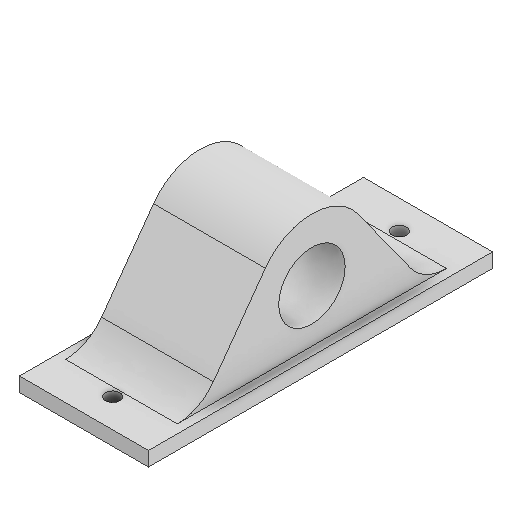
# Autodesk Inventor part: 8P - MainWing Joint
Saved by Autodesk Inventor 2025.1 (Build 291241000, 241)
## iProperties
Category: <PART CATAGORY>
Created: 2024-11-07
Part Number: 8P - MainWing Joint
Material: Generic
Document SubType Name: Modeling
Designer: alptl
Density: 1 g/cm^3
Appearance: Default
Title: <TITLE>
Author: alptl
Revision Number: 1
Autodesk Inventor part; units mm, degrees
ref_plane "YZ Plane" through (0, 0, 0) normal (1, 0, 0) x (0, 1, 0)
ref_plane "XZ Plane" through (0, 0, 0) normal (0, 1, 0) x (-1, 0, 0)
ref_plane "XY Plane" through (0, 0, 0) normal (0, 0, 1) x (1, 0, 0)
sketch "Sketch6" plane through (0, 0, 0) normal (0, 1, 0) x (-1, 0, 0)
  line L0 (22.5, 0) -> (22.5, -60)
  line L1 (22.5, -60) -> (-22.5, -60)
  line L2 (-22.5, -60) -> (-22.5, 0)
  circle A0 centre (0, -50) radius 2.5
  line L3 (-22.5, 0) -> (22.5, 0)
  point P0 (0, 0)
  dimension "d85" = 22.5
  dimension "d86" = 60
  dimension "d87" = 45
  dimension "d89" = 5
  constraints: 8 end point, 3 perpendicular, 1 centre point, 1 coincident
  measures "d85" distance of point (0, 0) L0.start
  measures "d86" distance of L0.start L0.end
  measures "d87" distance of L0.end L1.end
  measures "d89" diameter of A0
extrude "Extrusion3" add sketch "Sketch6" along normal blind 5
mirror "Mirror3" about plane through (-22.5, 0, 0) normal (0, 0, 1) of "Extrusion3"
sketch "Sketch7" plane through (0, 0, -60) normal (1, 0, 0) x (0, 0, -1)
  arc A0 (-43.7585, 36.671) -> (-76.2415, 36.671) centre (-60, 25) ccw
  circle A1 centre (-60, 23.3) radius 11.6
  line L0 (0, 5) -> (-120, 5) projected
  line L1 (-60, 5) -> (-99, 5)
  line L2 (-99, 5) -> (-76.2415, 36.671)
  line L3 (-60, 5) -> (-21, 5)
  line L4 (-21, 5) -> (-43.7585, 36.671)
  line L5 (-21, 5) -> (-99, 5)
  line L6 (-60, 17.6583) -> (-60, 50) construction
  line L7 (-120, 0) -> (0, 0) projected
  point P0 (-60, 0)
  point P1 (-60, 0)
  point P2 (-60, 0)
  dimension "d92" = 40
  dimension "d93" = 23.2
  dimension "d94" = 39
  dimension "d95" = 39
  dimension "d104" = 23.3
  dimension "d105" = 25
  constraints: 12 end point, 5 point on line, 4 midpoint, 2 centre point, 2 coincident, 2 point on circle, 2 tangent, 1 vertical
  measures "d92" diameter of A0
  measures "d93" diameter of A1
  measures "d94" distance of L1.start L1.end
  measures "d95" distance of L1.start L3.end
  measures "d104" distance of point (-60, 0) A1.centre
  measures "d105" distance of point (-60, 0) A0.centre
extrude "Extrusion6" add sketch "Sketch7" along normal mid plane 39
sketch "Sketch10" plane through (19.5, 0, -60) normal (1, 0, 0) x (0, 0, -1)
  circle A0 centre (-60, 23.3) radius 11.6 construction
  point P0 (-60, 0)
  constraints: 1 coincident
hole "Hole4" at (19.5, 23.3, 0) direction (-1, 0, 0) diameter 22.25 depth 7
sketch "Sketch11" plane through (-19.5, 0, -60) normal (-1, 0, 0) x (0, 0, 1)
  circle A0 centre (60, 23.3) radius 11.6 projected
  point P0 (60, 0)
  constraints: 1 coincident
hole "Hole5" at (-19.5, 23.3, 0) at (-19.5, 23.3, 0) direction (1, 0, 0) diameter 22.3 depth 7
fillet "Fillet1" radius 15.5 2 edges at (0, 5, 39) (0, 5, -39)
sketch "Sketch12" plane through (19.5, 36.671, -16.2415) normal (0, 0.5835502, -0.812077) x (-1, 0, 0)
  circle A0 centre (19.5, -5) radius 2.5
  point P0 (19.5, -20.3019)
  dimension "d121" = 5
  constraints: 1 centre point
  measures "d121" diameter of A0
extrude "Extrusion7" cut sketch "Sketch12" against normal blind 28.75
body "Solid2"
